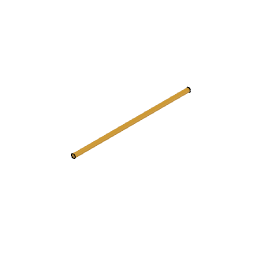
Long Bolt Front Side (Autodesk Fusion 360 design; units mm, degrees)
Autodesk Fusion 360 part; units mm, degrees
note: some values were not read from the file. Chosen so that the rebuilt part matches the saved one: which face or edge a step refers to.
sketch "Hole" plane through (0, 27, 0) normal (0, 1, 0) x (-1, 0, 0)
  circle A0 centre (-84, 10) radius 2
extrude "Extrude1" add sketch "Hole" against normal blind 15
extrude "Extrude2" add sketch "Hole" along normal blind 40
extrude "Extrude3" add 1 faces at (84.5374, 12, 9.8035) along direction (0, -1, 0) blind 40
extrude "Extrude4" cut 1 faces at (84.5374, -28, 9.8035) along direction (0, 1, 0) blind 40
extrude "Extrude5" cut 1 faces at (84.5374, 67, 9.8035) along direction (0, -1, 0) blind 40
extrude "Extrude6" add 1 faces at (84.5374, 27, 9.8035) along direction (0, 1, 0) blind 53
extrude "Extrude7" add 1 faces at (84.5374, 12, 9.8035) along direction (0, -1, 0) blind 50
named bodies: "Front Tube"
